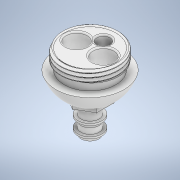
# Autodesk Inventor part: Lumipositor2-Bottom-V1
Saved by Autodesk Inventor 2022 (Build 260153000, 153)
## iProperties
Created: 2021-10-25
Part Number: Lumipositor2-Bottom-V1
Material: PC/ABS Plastic
Document SubType Name: Modeling
Designer: incep
Density: 0.357273 g/cm^3
Appearance: Smooth - White
Author: incep
## iProperties of the stored document Lumipositor2-Bottom-V1_3DPrint.ipt
Created: 2021-10-27
Part Number: Lumipositor2-Bottom-V1_3DPrint
Material: Generic
Document SubType Name: Modeling
Designer: incep
Density: 1 g/cm^3
Appearance: Default
Author: incep
Autodesk Inventor part; units mm, degrees
ref_plane "YZ Plane" through (0, 0, 0) normal (1, 0, 0) x (0, 1, 0)
ref_plane "XZ Plane" through (0, 0, 0) normal (0, 1, 0) x (-1, 0, 0)
sketch "Sketch2" plane through (0, 0, 0) normal (0, 0, 1) x (1, 0, 0)
  line L0 (0, 0) -> (15, 0)
  line L1 (15, 0) -> (15, -6.2)
  line L2 (14, -10) -> (17.8115, -10)
  arc A0 (4.7625, -22.8765) -> (17.8115, -10) centre (0, -5) ccw
  line L3 (0, -22.8765) -> (4.7625, -22.8765) construction
  line L4 (4.7625, -22.8765) -> (4.7625, -38.8765) construction
  line L5 (4.7625, -38.8765) -> (0, -38.8765) construction
  line L6 (0, -38.8765) -> (0, -22.8765) construction
  line L7 (3.0125, -38.8765) -> (3.0125, -22.8765) construction
  line L8 (4.7625, -35.8765) -> (6.2625, -35.8765) construction
  line L9 (6.2625, -35.8765) -> (6.2625, -38.8765) construction
  line L10 (6.2625, -38.8765) -> (4.7625, -38.8765) construction
  line L11 (4.7625, -38.8765) -> (4.7625, -35.8765) construction
  line L12 (4.7625, -32.8765) -> (6.2625, -32.8765) construction
  line L13 (6.2625, -32.8765) -> (6.2625, -35.8765) construction
  line L14 (6.2625, -35.8765) -> (4.7625, -35.8765) construction
  line L15 (4.7625, -35.8765) -> (4.7625, -32.8765) construction
  line L16 (4.7625, -29.8765) -> (6.2625, -29.8765) construction
  line L17 (6.2625, -29.8765) -> (6.2625, -32.8765) construction
  line L18 (6.2625, -32.8765) -> (4.7625, -32.8765) construction
  line L19 (4.7625, -32.8765) -> (4.7625, -29.8765) construction
  line L20 (3.0125, -38.8765) -> (4.7625, -38.8765)
  line L21 (4.7625, -38.8765) -> (6.2625, -36.8765)
  line L22 (6.2625, -35.8765) -> (6.2625, -36.8765)
  line L23 (6.2625, -35.8765) -> (4.7625, -35.8765)
  line L24 (4.7625, -35.8765) -> (4.7625, -32.8765)
  line L25 (6.2625, -29.8765) -> (4.7625, -29.8765)
  line L26 (4.7625, -29.8765) -> (4.7625, -22.8765)
  line L27 (4.7625, -32.8765) -> (6.2625, -30.8765)
  line L28 (6.2625, -30.8765) -> (6.2625, -29.8765)
  line L29 (3.0125, -38.8765) -> (3.0125, -20.8765)
  line L30 (0, -14) -> (17.8115, -14) construction
  line L31 (3.0125, -20.8765) -> (9, -14)
  line L32 (17.8115, -10) -> (17.8115, -14) construction
  line L33 (9, -14) -> (0, -14)
  line L34 (0, 0) -> (0, -14)
  line L35 (14, -10) -> (13.5, -10)
  line L36 (13.5, -10) -> (13.5, -6.2)
  line L37 (13.5, -6.2) -> (15, -6.2)
  circle A1 centre (0, -5) radius 18 construction
  line L38 (18, -5) -> (-18, -5) construction
  line L39 (-18, -5) -> (-18, 55) construction
  line L40 (-18, 55) -> (18, 55) construction
  line L41 (18, 55) -> (18, -5) construction
  circle A2 centre (0, 55) radius 18 construction
  dimension "d68" = 36
  dimension "d71" = 36
  dimension "d17" = 1.5
  dimension "d18" = 3
  dimension "d19" = 7
  dimension "d20" = 4.7625
  dimension "d21" = 1.75
  dimension "d22" = 1
  dimension "d24" = 2
  dimension "d31" = 5
  dimension "d32" = 3.8
  dimension "d34" = 4
  dimension "d35" = 10
  dimension "d36" = 15
  dimension "d69" = 18.5
  dimension "d70" = 60
  dimension "d72" = 5
  dimension "d86" = 13.5
  dimension "d87" = 9
  constraints: 84 end point, 11 parallel, 11 perpendicular, 9 collinear, 8 horizontal, 7 point on line, 2 horizontal alignment, 2 point on circle, 2 vertical, 1 centre point, 1 coincident, 1 midpoint, 1 vertical alignment, 4 other
  measures "d17" distance of L4.end L9.end
  measures "d18" distance of L8.end L9.end
  measures "d19" distance from line of L3.end L16
  measures "d20" distance of L4.end L5.end
  measures "d21" distance of L4.end L7.start
  measures "d22" distance of L8.end L21.end
  measures "d24" distance from line of L3 L29.end
  measures "d31" distance from line of L2 A0.centre
  measures "d32" distance of L35.end L36.end
  measures "d34" distance between parallel lines of L33 L2
  measures "d35" distance from line of L0.end L2
  measures "d36" distance from line of L0.start L1
  measures "d69" radius of A0
  measures "d70" distance of L38.end L39.end
  measures "d72" distance of A0.centre L0.start
  measures "d86" distance between parallel lines of L36 L34
  measures "d87" distance of L31.end L30.start
revolve "Revolution1" add sketch "Sketch2" angle 360 about axis through (0, 0, 0) along (0, -1, 0)
sketch "Sketch3" plane through (0, 0, 0) normal (0, 1, 0) x (1, 0, 0)
  circle A0 centre (-7, 0) radius 5.5
  circle A1 centre (7, 0) radius 5.5
  line L0 (-7, 0) -> (7, 0) construction
  circle A2 centre (0, 7) radius 3.5
  point P0 (0, 0)
  point P1 (0, 0)
  dimension "d37" = 11
  dimension "d38" = 14
  dimension "d39" = 7
  dimension "d40" = 7
  constraints: 3 centre point, 2 end point, 1 coincident, 1 equal radius, 1 horizontal, 1 midpoint
  measures "d37" diameter of A0
  measures "d38" distance of L0.start L0.end
  measures "d39" diameter of A2
  measures "d40" distance of A2.centre point (0, 0)
extrude "Extrusion2" cut sketch "Sketch3" against normal blind 10
thread "Thread1" size "M30x2" class "6g" standard "ANSI Metric M Profile" full length
sketch "Sketch7" plane through (0, 0, 0) normal (0, 0, 1) x (1, 0, 0)
  arc A0 (-18, -5) -> (18, -5) centre (0, -5) ccw
  line L0 (18, -5) -> (18, 55)
  line L1 (-18, 55) -> (-18, -5)
  arc A1 (18, 55) -> (-18, 55) centre (0, 55) ccw
  line L2 (0, 73) -> (0, -23)
  point P0 (0, 0)
  dimension "d73" = 36
  dimension "d74" = 5
  dimension "d76" = 60
  constraints: 6 end point, 6 point on circle, 3 tangent, 2 centre point, 2 parallel, 1 point on line, 1 vertical
  measures "d73" diameter of A0
  measures "d74" distance of A0.centre point (0, 0)
  measures "d76" distance of L0.start L0.end
revolve "Revolution4" [suppressed]
sketch "Sketch8" plane through (-7, -10, 0) normal (0, 1, 0) x (1, 0, 0)
  circle A0 centre (0, 0) radius 1
  circle A1 centre (14, 0) radius 1
  circle A2 centre (7, 7) radius 1
  circle A3 centre (0, 0) radius 1.268
  circle A4 centre (7, 7) radius 1.268
  circle A5 centre (14, 0) radius 1.268
  line L0 (0, 0) -> (14, 0) construction
  line L1 (7, 7) -> (7, 0) construction
  dimension "d78" = 2
  dimension "d79" = 2.536
  dimension "d80" = 14
  dimension "d81" = 7
  constraints: 6 centre point, 4 coincident, 4 end point, 4 equal radius, 1 horizontal, 1 midpoint, 1 vertical
  measures "d78" diameter of A0
  measures "d79" diameter of A3
  measures "d80" distance of A1.centre A0.centre
  measures "d81" distance of L1.start L1.end
extrude "Extrusion3" cut sketch "Sketch8" against normal blind 0.635 contours A0 | A1 | A2 | A3 | A4 | A5
extrude "Extrusion4" cut sketch "Sketch8" against normal blind 5 contours A0 | A1 | A2
ref_plane "Work Plane1" through (0, -23.8765, 0) normal (0, 1, 0) x (1, 0, 0)
sketch "Sketch9" plane through (0, -23.8765, 0) normal (0, 1, 0) x (1, 0, 0)
  line L0 (-8, 4.6188) -> (0, 9.2376)
  line L1 (0, 9.2376) -> (8, 4.6188)
  line L2 (8, 4.6188) -> (8, -4.6188)
  line L3 (8, -4.6188) -> (0, -9.2376)
  line L4 (0, -9.2376) -> (-8, -4.6188)
  line L5 (-8, -4.6188) -> (-8, 4.6188)
  circle A0 centre (0, 0) radius 4
  dimension "d89" = 8
  dimension "d90" = 8
  constraints: 12 end point, 2 coincident, 1 centre point, 13 other
  measures "d89" distance from line of L5 point (0, 0)
  measures "d90" diameter of A0
extrude "Extrusion5" add sketch "Sketch9" along normal blind 3
fillet "Fillet1" radius 0.75 10 edges at (-4, -23.8765, 6.9282) (4, -23.8765, 6.9282) (-8, -23.8765, 0) (-4, -23.8765, -6.9282) (4, -23.8765, -6.9282) (8, -23.8765, 0) (-4.7625, -23.8765, 0) (-3.5, 0, -7) (-12.5, 0, 0) (1.5, 0, 0)
sketch "Sketch11" plane through (0, -6.2, 0) normal (-1, 0, 0) x (0, 0, 1)
  line L0 (15, 0) -> (15, 6.2)
  line L1 (15, 6.2) -> (13.5171, 6.2)
  line L2 (13.5171, 6.2) -> (13.5171, 0)
  line L3 (13.5171, 0) -> (15, 0)
  line L4 (0, -1.24) -> (0, 7.44) projected
  constraints: 8 end point
revolve "Revolution5" cut sketch "Sketch11" angle 360 about axis through (0, -6.2, 0) along (0, 1, 0)
sketch "Sketch12" plane through (0, -6.2, 0) normal (-1, 0, 0) x (0, 0, 1)
  line L0 (15, 0) -> (15, 6.2)
  line L1 (15, 6.2) -> (13.5171, 6.2)
  line L2 (13.5171, 6.2) -> (13.5171, 0)
  line L3 (13.5171, 0) -> (15, 0)
  line L4 (0, -1.24) -> (0, 7.44) projected
  constraints: 8 end point
revolve "Revolution6" add sketch "Sketch12" angle 360 about axis through (0, -6.2, 0) along (0, 1, 0) separate body
sketch "Sketch10" plane through (0, -6.2, 0) normal (1, 0, 0) x (0, 1, 0)
  line L0 (-1.1668, -13.6184) -> (-1.0001, -13.6184) construction
  line L1 (0.1666, -14.899) -> (-0.0001, -15.2192) construction
  line L2 (-2.0001, -15.2192) -> (-2.1668, -14.899) construction
  line L3 (-0.8334, -13.6184) -> (-1.0001, -13.2982) construction
  line L4 (-1.0001, -13.2982) -> (-1.1668, -13.6184) construction
  line L5 (-2.0001, -15.2192) -> (-1.8334, -14.899) construction
  line L6 (-0.8334, -13.6184) -> (-0.1668, -14.899)
  line L7 (-2.1668, -14.899) -> (-1.8334, -14.899) construction
  arc A0 (-2.1668, -14.899) -> (-2.0001, -15.0002) centre (-2.0001, -14.8123) ccw construction
  line L8 (0.1666, -14.899) -> (-0.1668, -14.899) construction
  line L9 (-2.0001, -15.2192) -> (-2.0001, -14.899) construction
  line L10 (-0.0001, -15.2192) -> (-0.0001, -14.899) construction
  line L11 (-1.0001, -13.2982) -> (-1.0001, -13.5172) construction
  line L12 (-2.0001, -15.0002) -> (-0.0001, -15.0002)
  arc A1 (-2.0001, -15.0002) -> (-1.8334, -14.899) centre (-2.0001, -14.8123) ccw
  line L13 (-0.1668, -14.899) -> (-0.0001, -15.2192) construction
  line L14 (-1.8334, -14.899) -> (-1.1668, -13.6184)
  line L15 (-0.0001, -0.0002) -> (-0.0001, 0.0177)
  line L16 (-0.0001, 0.0177) -> (-0.0001, -0.0002)
  line L17 (-0.0001, -0.0002) -> (0.0334, -0.0002)
  arc A2 (-0.1668, -14.899) -> (-0.0001, -15.0002) centre (-0.0001, -14.8123) ccw
  arc A3 (-0.0001, -15.0002) -> (0.1666, -14.899) centre (-0.0001, -14.8123) ccw construction
  arc A4 (-1.0001, -13.5172) -> (-1.1668, -13.6184) centre (-1.0001, -13.7051) ccw
  arc A5 (-0.8334, -13.6184) -> (-1.0001, -13.5172) centre (-1.0001, -13.7051) ccw
  line L18 (-1.0001, -13.5172) -> (-1.0001, -13.6184) construction
  line L19 (-1.0001, -13.6184) -> (-0.8334, -13.6184) construction
  dimension "d94" = 55
  dimension "d95" = 0.3202
  dimension "d96" = 0.3202
  dimension "Sketch10_ThreadOffset" = 0
  dimension "Sketch10_MajorRadius" = 15
  dimension "d99" = 2
  dimension "Sketch10_MinorRadius" = 13.5171
  constraints: 40 end point, 12 point on circle, 10 parallel, 8 tangent, 6 centre point, 6 collinear, 2 midpoint, 2 point on line, 1 horizontal, 1 perpendicular, 3 other
  measures "d94" angle of L6 L14
  measures "d95" distance of L3.end L0.end
  measures "d96" distance of L1.end L10.end
  measures "Sketch10_ThreadOffset" distance between parallel lines of L15 L10
  measures "Sketch10_MajorRadius" distance from line of L12 L15.start
  measures "d99" distance from line of L1.end L9
  measures "Sketch10_MinorRadius" distance edge to line of A5 L17
coil "Coil2" sketch "Sketch10" operation cut axis through (0, -6.2, 0) along (0, 1, 0) pitch 2.002 turns 5.094905 hand right bodies 2
equation "\"d54\" = 0.25"
equation "\"Sketch4_Pitch\" = 2"
equation "\"d56\" = 60deg"
equation "\"d101\" = 55deg"
equation "\"Sketch10_Pitch\" = 2"
body "Solid2"
body "Solid4"
body "Solid5"
